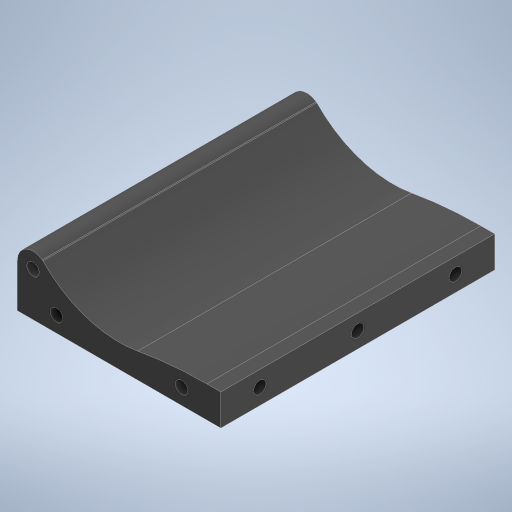
# Autodesk Inventor part: hipjoint_toleg_middle
Saved by Autodesk Inventor 2024.1 (Build 281209000, 209)
## iProperties
Created: 2024-02-12
Part Number: hipjoint_toleg_middle
Material: 一般
Document SubType Name: Modeling
Designer: hibik
Density: 1 g/cm^3
Appearance: 既定
Author: hibik
Autodesk Inventor part; units mm, degrees
ref_plane "YZ Plane" through (0, 0, 0) normal (1, 0, 0) x (0, 1, 0)
ref_plane "XZ Plane" through (0, 0, 0) normal (0, 1, 0) x (-1, 0, 0)
ref_plane "XY Plane" through (0, 0, 0) normal (0, 0, 1) x (1, 0, 0)
sketch "スケッチ1" plane through (0, 0, 0) normal (0, 0, 1) x (1, 0, 0)
  line L0 (0, 16.5) -> (26, 16.5)
  line L1 (26, 16.5) -> (26, 0)
  line L2 (26, 0) -> (0, 0)
  line L3 (0, 0) -> (0, 16.5)
  circle A0 centre (13, 16.5) radius 12.5
  line L4 (13, 4) -> (26, 4)
  arc A1 (0, 10.25) -> (13, 4) centre (13, 20.645) ccw
  line L5 (13, 4) -> (0, 4)
  point P0 (25.5, 16.5)
  point P1 (0.5, 16.5)
  dimension "d0" = 25
  dimension "d1" = 26
  dimension "d2" = 16.5
  dimension "d8" = 6.25
  dimension "d9" = 6.25
  constraints: 12 end point, 3 horizontal, 3 point on line, 2 parallel, 2 perpendicular, 2 point on circle, 1 centre point, 1 coincident, 1 midpoint, 1 tangent, 3 other
  measures "d1" distance of L0.start L0.end
  measures "d2" distance of L2.end L0.start
  measures "d8" distance of L5.end A1.start
  measures "d9" distance of L0.start A1.start
extrude "押し出し1" add sketch "スケッチ1" along normal blind 35 contours L5 L3 A1 | L4 L1 L2 L3 L5
fillet "フィレット4" radius 2 1 edges at (0, 10.25, 17.5)
sketch "スケッチ2" plane through (26, 0, 0) normal (1, 0, 0) x (0, 0, -1)
  circle A0 centre (-30, 2) radius 0.8
  circle A1 centre (-5, 2) radius 0.8
  line L0 (0, 0) -> (-35, 0) projected
  line L1 (-35, 0) -> (-35, 4) projected
  line L2 (0, 0) -> (0, 4) projected
  circle A2 centre (-17.5, 2) radius 0.8
  dimension "d11" = 1.6
  dimension "d12" = 1.6
  dimension "d13" = 2
  dimension "d14" = 5
  dimension "d15" = 5
  dimension "d26" = 12.5
  dimension "d27" = 12.5
  constraints: 3 centre point, 2 horizontal alignment, 1 equal radius
  measures "d11" diameter of A0
  measures "d12" diameter of A1
  measures "d13" distance from line of L0 A0.centre
  measures "d14" distance from line of L1 A0.centre
  measures "d15" distance from line of L2 A1.centre
  measures "d26" distance of A2.centre A0.centre
  measures "d27" distance of A2.centre A1.centre
extrude "押し出し2" cut sketch "スケッチ2" against normal through all
sketch "スケッチ3" plane through (0, 0, 35) normal (0, 0, 1) x (1, 0, 0)
  circle A0 centre (2, 5.5906) radius 0.8
  circle A1 centre (5, 2) radius 0.8
  circle A2 centre (21, 2) radius 0.8
  line L0 (0, 0) -> (26, 0) projected
  line L1 (26, 0) -> (26, 4) projected
  line L2 (0, 5.5906) -> (0, 0) projected
  arc A3 (3.1799, 7.2054) -> (0, 5.5906) centre (2, 5.5906) ccw projected
  dimension "d18" = 1.6
  dimension "d19" = 1.6
  dimension "d20" = 1.6
  dimension "d21" = 2
  dimension "d22" = 5
  dimension "d23" = 5
  constraints: 3 centre point, 1 concentric, 1 horizontal alignment
  measures "d18" diameter of A0
  measures "d19" diameter of A1
  measures "d20" diameter of A2
  measures "d21" distance from line of L0 A1.centre
  measures "d22" distance from line of L1 A2.centre
  measures "d23" distance from line of L2 A1.centre
extrude "押し出し3" cut sketch "スケッチ3" against normal through all
sketch "スケッチ4" plane through (0, 0, 35) normal (0, 0, 1) x (1, 0, 0)
  arc A0 (3.1799, 7.2054) -> (13, 4) centre (13, 20.645) ccw projected
  circle A1 centre (13, 16.5) radius 12.5 construction
  line L0 (13, 16.5) -> (13, 4) construction
  circle A2 centre (13, 16.5) radius 13.5
  point P0 (0, 0)
  dimension "d30" = 25
  dimension "d31" = 27
  constraints: 2 end point, 1 centre point, 1 coincident, 1 vertical, 1 vertical alignment, 3 other
  measures "d31" diameter of A2
extrude "押し出し4" cut sketch "スケッチ4" against normal through all
fillet "フィレット5" radius 50 1 edges at (18.099, 4, 17.5)
equation "\"d8\" = d9"
equation "\"d26\" = d27"
